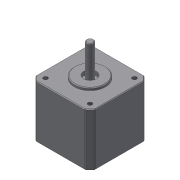
# Autodesk Inventor part: Stepper Motor
Saved by Autodesk Inventor 2015 (Build 190159000, 159)
## iProperties
Created: 2020-01-08
Part Number: Stepper Motor
Material: Generic
Document SubType Name: Modeling
Designer: Ghassan Yusuf
Density: 1 g/cm^3
Appearance: Default
Author: Ghassan Yusuf
Autodesk Inventor part; units mm, degrees
ref_plane "YZ Plane" through (0, 0, 0) normal (1, 0, 0) x (0, 1, 0)
ref_plane "XZ Plane" through (0, 0, 0) normal (0, 1, 0) x (-1, 0, 0)
ref_plane "XY Plane" through (0, 0, 0) normal (0, 0, 1) x (1, 0, 0)
sketch "Sketch1" plane through (0, 0, 0) normal (0, 0, 1) x (1, 0, 0)
  line L0 (-17.4645, 21) -> (17.4645, 21)
  line L1 (21, 17.4645) -> (21, -17.4645)
  line L2 (17.4645, -21) -> (-17.4645, -21)
  line L3 (-21, -17.4645) -> (-21, 17.4645)
  line L4 (-21, 17.4645) -> (-17.4645, 21)
  line L5 (-21, 17.4645) -> (-16, 17.4645) construction
  line L6 (-17.4645, -21) -> (-21, -17.4645)
  line L7 (21, -17.4645) -> (17.4645, -21)
  line L8 (17.4645, 21) -> (21, 17.4645)
  point P0 (0, 0)
  point P1 (0, 21)
  point P2 (-21, 0)
  dimension "d4" = 360
  dimension "d1" = 45
  dimension "d6" = 5
  dimension "d7" = 42
  dimension "d8" = 42
  constraints: 18 end point, 5 point on line, 2 coincident, 2 horizontal, 2 midpoint, 2 parallel, 1 equal length, 1 horizontal alignment, 1 perpendicular, 1 vertical alignment, 13 other
  measures "d1" angle of L5 L4
  measures "d6" distance of L0.start L3.end
  measures "d7" distance between parallel lines of L2 L0
  measures "d8" distance between parallel lines of L1 L3
extrude "Extrusion1" add sketch "Sketch1" along normal blind 37.5
sketch "Sketch2" plane through (0, 0, 37.5) normal (0, 0, 1) x (1, 0, 0)
  circle A0 centre (0, 0) radius 11
  dimension "d11" = 22
  constraints: 1 centre point, 1 coincident
  measures "d11" diameter of A0
extrude "Extrusion2" add sketch "Sketch2" along normal blind 1.8
sketch "Sketch3" plane through (0, 0, 39.3) normal (0, 0, 1) x (1, 0, 0)
  circle A0 centre (0, 0) radius 4.6
  dimension "d14" = 9.2
  constraints: 1 centre point, 1 coincident
  measures "d14" diameter of A0
extrude "Extrusion3" cut sketch "Sketch3" against normal blind 3
sketch "Sketch4" plane through (0, 0, 36.3) normal (0, 0, 1) x (1, 0, 0)
  circle A0 centre (0, 0) radius 2.5
  dimension "d17" = 5
  constraints: 1 centre point, 1 coincident
  measures "d17" diameter of A0
extrude "Extrusion4" add sketch "Sketch4" along normal blind 24
sketch "Sketch5" plane through (0, 0, 60.3) normal (0, 0, 1) x (1, 0, 0)
  arc A0 (-2.25, 1.0897) -> (-2.25, -1.0897) centre (0, 0) ccw
  line L0 (-2.25, 1.0897) -> (-2.25, -1.0897)
  circle A1 centre (0, 0) radius 2.5 projected
  dimension "d20" = 2.25
  constraints: 2 end point, 2 point on circle, 1 centre point, 1 coincident, 1 concentric, 1 vertical
  measures "d20" distance from line of point (0, 0) L0
extrude "Extrusion5" cut sketch "Sketch5" against normal blind 21 contours L0 A0
chamfer "Chamfer1" distance 0.5 angle 45 2 edges at (0.559, -2.4367, 60.3) (0.559, 2.4367, 60.3)
sketch "Sketch6" plane through (0, 0, 37.5) normal (0, 0, 1) x (1, 0, 0)
  circle A0 centre (-15.8, 15.8) radius 1.5
  circle A1 centre (15.8, 15.8) radius 1.5
  circle A2 centre (-15.8, -15.8) radius 1.5
  circle A3 centre (15.8, -15.8) radius 1.5
  point P0 (0, 0)
  dimension "d27" = 15.8
  dimension "d28" = 31.6
  dimension "d29" = 15.8
  dimension "d30" = 31.6
  dimension "d31" = 3
  constraints: 4 centre point, 3 equal radius, 2 horizontal alignment, 2 vertical alignment
  measures "d27" horizontal distance of point (0, 0) A0.centre
  measures "d28" distance of A2.centre A0.centre
  measures "d29" horizontal distance of point (0, 0) A0.centre
  measures "d30" distance of A1.centre A0.centre
  measures "d31" diameter of A0
extrude "Extrusion6" cut sketch "Sketch6" against normal blind 5
thread "Thread1" size "M3x0.5" class "6H" standard "ANSI Metric M Profile" full length
thread "Thread2" size "M3x0.5" class "6H" standard "ANSI Metric M Profile" full length
thread "Thread3" size "M3x0.5" class "6H" standard "ANSI Metric M Profile" full length
thread "Thread4" size "M3x0.5" class "6H" standard "ANSI Metric M Profile" full length
chamfer "Chamfer2" distance 0.5 angle 45 1 edges at (-11, 0, 39.3)
chamfer "Chamfer3" distance 0.5 angle 45 24 edges at (0, -21, 0) (19.2322, -19.2322, 0) (21, 0, 0) (-21, 0, 0) (0, 21, 0) (21, 0, 37.5) (0, 21, 37.5) (-21, 0, 37.5) (0, -21, 37.5) (19.2322, 19.2322, 37.5) (-19.2322, -19.2322, 37.5) (19.2322, -19.2322, 37.5) (17.4645, -21, 18.75) (21, -17.4645, 18.75) (-17.4645, -21, 18.75) (-21, -17.4645, 18.75) (21, 17.4645, 18.75) (17.4645, 21, 18.75) (-17.4645, 21, 18.75) (-21, 17.4645, 18.75) (-19.2322, 19.2322, 0) (-19.2322, -19.2322, 0) (19.2322, 19.2322, 0) (-19.2322, 19.2322, 37.5)
equation "\"d27\" = 0.5 * d28"
equation "\"d29\" = d27"
equation "\"d30\" = d28"
body "Solid1"
